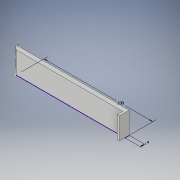
# Autodesk Inventor part: Hebel_Klemme_oben
Saved by Autodesk Inventor 2018 (Build 220112000, 112)
## iProperties
Created: 2018-02-02
Part Number: Hebel_Klemme_oben
Material: Generisch
Document SubType Name: Modeling
Designer: Julian
Density: 1 g/cm^3
Appearance: Vorgabe
Mass: 8.3135 g
Surface Area: 53.4214 cm^2
Volume: 8.3135 cm^3
Author: Julian
Autodesk Inventor part; units mm, degrees
ref_plane "YZ Plane" through (0, 0, 0) normal (1, 0, 0) x (0, 1, 0)
ref_plane "XZ Plane" through (0, 0, 0) normal (0, 1, 0) x (-1, 0, 0)
ref_plane "XY Plane" through (0, 0, 0) normal (0, 0, 1) x (1, 0, 0)
sketch "Skizze1" plane through (0, 0, 0) normal (0, 0, 1) x (1, 0, 0)
  line L0 (0, 0) -> (100, 0)
  line L1 (100, 0) -> (100, 4)
  line L2 (100, 4) -> (0, 4)
  line L3 (0, 4) -> (0, 0)
  dimension "d0" = 100
  dimension "d1" = 4
  constraints: 8 end point, 2 parallel, 1 horizontal, 1 perpendicular
  measures "d0" distance of L1.end L2.end
  measures "d1" distance between parallel lines of L2 L0
extrude "Extrusion1" add sketch "Skizze1" along normal blind 20
sketch "Skizze2" plane through (0, 0, 0) normal (0, 0, -1) x (-1, 0, 0)
  line L0 (0, 4) -> (0, 0) projected
  line L1 (-100, 4) -> (0, 4) projected
  line L2 (0, 4) -> (2.5, 4) construction
  line L3 (1.7678, 5.7678) -> (1.7678, 5.75)
  arc A0 (2.8969, 2.663) -> (0.0178, 4) centre (1.7678, 4) ccw
  line L4 (0, 0) -> (3.0052, 2.7626)
  line L5 (0, 4) -> (0.0179, 4.0179)
  line L6 (1.7499, 5.7499) -> (1.7678, 5.7678)
  circle A1 centre (1.7678, 4) radius 0.75
  dimension "d4" = 2.5
  dimension "d6" = 3.5
  dimension "d9" = 1.5
  constraints: 10 end point, 6 point on circle, 2 centre point, 2 point on line, 1 coincident, 1 horizontal, 1 perpendicular
  measures "d4" distance of L0.start L3.start
  measures "d6" diameter of A0
  measures "d9" diameter of A1
extrude "Extrusion2" add sketch "Skizze2" against normal blind 20 contours L5 A0 L4 L0 | A1
sketch "Skizze3" plane through (0, 0, 0) normal (0, 0, -1) x (-1, 0, 0)
  point P0 (0, 0)
extrude "Extrusion3" cut sketch "Skizze2" against normal blind 20 contours A1
sketch "Skizze4" plane through (100, 0, 0) normal (0, -1, 0) x (1, 0, 0)
  line L0 (0, 20) -> (-100, 20) projected
  line L1 (0, 0) -> (-100, 0) projected
  line L2 (0, 20) -> (-2, 20)
  line L3 (-2, 20) -> (-2, 0)
  line L4 (-2, 0) -> (0, 0)
  line L5 (0, 0) -> (0, 20)
  dimension "d12" = 2
  constraints: 8 end point, 2 parallel, 1 horizontal, 1 perpendicular, 1 point on line
  measures "d12" distance of L4.end L3.end
extrude "Extrusion4" add sketch "Skizze4" along normal blind 5
sketch "Skizze6" plane through (0, 0, 0) normal (0, -1, 0) x (1, 0, 0)
  line L0 (0, 0) -> (0, 20) projected
  line L1 (0, 20) -> (0, 15)
  line L2 (0, 15) -> (0, 10)
  line L3 (0, 10) -> (0, 5)
  line L4 (0, 5) -> (0, 0)
  line L5 (-3.5178, 0) -> (-0.0179, 0) projected
  line L6 (0, 0) -> (-3.5178, 0)
  line L7 (-3.5178, 0) -> (-3.5178, 5)
  line L8 (-3.5178, 0) -> (-3.5178, 20) projected
  line L9 (0, 5) -> (-3.5178, 5)
  line L10 (0, 15) -> (-3.5178, 15)
  line L11 (-3.5178, 15) -> (-3.5178, 10)
  line L12 (0, 10) -> (-3.5178, 10)
  point P0 (-3.0052, 0)
  dimension "d22" = 5
  dimension "d23" = 5
  dimension "d24" = 5
  constraints: 20 end point, 5 point on line, 3 perpendicular, 1 collinear, 1 midpoint, 1 parallel
  measures "d22" distance of L0.end L1.end
  measures "d23" distance of L1.end L2.end
  measures "d24" distance of L2.end L3.end
extrude "Extrusion5" cut sketch "Skizze6" against normal blind 50 contours L6 L5 L7 L9 L0 | L12 L8 L10 L0
